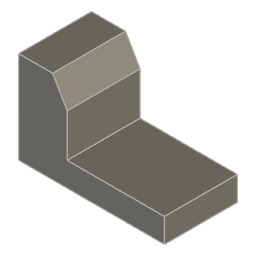
irtxcase (Autodesk Fusion 360 archive; units mm, degrees)
design "PCBMount - non-clip - 1mm"
Autodesk Fusion 360 part; units mm, degrees
note: some values were not read from the file. Chosen so that the rebuilt part matches the saved one: which face or edge a step refers to; which pieces of a blend or face edit are solid. Set by a fixed rule: which sketch regions a step uses.
sketch "Sketch1" plane through (0, 0, 0) normal (0, 1, 0) x (1, 0, 0)
  line L0 (0, 0) -> (6, 0)
  line L1 (6, 0) -> (6, -1)
  line L2 (6, -1) -> (2, -1)
  line L3 (2, -1) -> (2, -3.8)
  line L4 (2, -3.8) -> (0, -3.8)
  line L5 (0, -3.8) -> (0, 0)
  dimension "d1" = 2.8
  dimension "d2" = 1
  dimension "d3" = 2
  dimension "d4" = 4
  constraint coincident L0.start L5.end
  constraint horizontal L0
  constraint perpendicular L0 L1
  constraint perpendicular L1 L2
  constraint perpendicular L2 L3
  constraint perpendicular L4 L5
  constraint coincident L3.end L4.start
  measures "d1" distance of L2.end L3.end
  measures "d2" distance of L0.end L1.end
  measures "d3" distance of L3 L5
  measures "d4" distance of L1 L3
extrude "Extrude1" add sketch "Sketch1" along normal blind 3
sketch "Sketch4" plane through (0, 0, 0) normal (0, 0, -1) x (1, 0, 0)
  line L0 (6, 0) -> (0, 0)
  line L1 (0, 0) -> (0, -3)
  line L2 (0, -3) -> (6, -3)
  line L3 (6, -3) -> (6, 0)
  line L4 (0, -1.5) -> (6, -1.5) construction
  line L5 (2, 0) -> (2, -3) construction
  point P0 (2, -1.5)
  constraint midpoint L1 L4.start
  constraint midpoint L3 L4.end
  constraint midpoint L5 P0
chamfer "Chamfer3" distance 0.6 angle 60 1 edges at (2, 1.5, 3.8) measured on face at (1.3333, 1, 3.8)

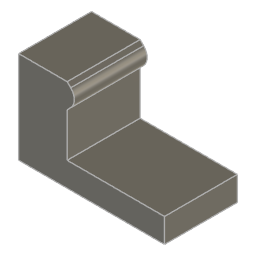
design "PCBMount - 1mm"
Autodesk Fusion 360 part; units mm, degrees
sketch "Sketch1" plane through (0, 0, 0) normal (0, 1, 0) x (1, 0, 0)
  line L0 (0, 0) -> (6, 0)
  line L1 (6, 0) -> (6, -1)
  line L2 (6, -1) -> (2, -1)
  line L3 (2, -1) -> (2, -2.8)
  line L4 (2, -2.8) -> (2.5, -2.8)
  line L5 (2.5, -2.8) -> (2.5, -3.8)
  line L6 (2.5, -3.8) -> (0, -3.8)
  line L7 (0, -3.8) -> (0, 0)
  dimension "d1" = 1.8
  dimension "d2" = 1
  dimension "d3" = 2
  dimension "d4" = 4
  dimension "d5" = 1
  dimension "d6" = 0.5
  constraint coincident L0.start L7.end
  constraint horizontal L0
  constraint perpendicular L0 L1
  constraint perpendicular L1 L2
  constraint perpendicular L2 L3
  constraint perpendicular L3 L4
  constraint perpendicular L4 L5
  constraint perpendicular L5 L6
  constraint perpendicular L6 L7
  measures "d1" distance of L2.end L3.end
  measures "d2" distance of L0.end L1.end
  measures "d3" distance of L3 L7
  measures "d4" distance of L1 L3
  measures "d5" distance of L4.end L5.end
  measures "d6" distance of L3 L5
extrude "Extrude1" add sketch "Sketch1" along normal blind 3
sketch "Sketch2" plane through (0, 0, 1) normal (0, 0, 1) x (-1, 0, 0)
  line L0 (-2, 0) -> (-6, 0)
  line L1 (-6, 0) -> (-6, -3)
  line L2 (-6, -3) -> (-2, -3)
  line L3 (-2, -3) -> (-2, 0)
  line L4 (0, 0) -> (0, -3) construction
  line L5 (-6, -1.5) -> (0, -1.5) construction
  line L6 (-4.5, -3) -> (-4.5, 0) construction
  line L7 (-6, 0) -> (-2, 0) construction
  circle A0 centre (-4.5, -1.5) radius 1.25
  dimension "d9" = 1.5
  dimension "d10" = 1.5
  dimension "d11" = 2.5
  dimension "d15" = 2.5
  constraint midpoint L1 L5.start
  constraint midpoint L4 L5.end
  constraint coincident L2 L6.start
  constraint coincident L0 L6.end
  constraint perpendicular L6 L7
  constraint midpoint L6 A0.centre
  measures "d9" distance of L5 L7
  measures "d10" distance of L1 L6
  measures "d11" diameter of A0
  measures "d15" distance of L3 L6
chamfer "Chamfer2" distance 0.5 angle 45 2 edges at (2.5, 1.5, 2.8) (2.5, 1.5, 3.8)
fillet "Fillet1" radius 0.5 4 edges at (2.5, 0, 3.3) (2.5, 1.5, 3.2999) (2.5, 3, 3.3) (2.5, 1.5, 3.3001)
sketch "Sketch4" plane through (0, 0, 0) normal (0, 0, -1) x (1, 0, 0)
  line L0 (6, 0) -> (0, 0)
  line L1 (0, 0) -> (0, -3)
  line L2 (0, -3) -> (6, -3)
  line L3 (6, -3) -> (6, 0)
  line L4 (0, -1.5) -> (6, -1.5) construction
  line L5 (2, 0) -> (2, -3) construction
  point P0 (2, -1.5)
  constraint midpoint L1 L4.start
  constraint midpoint L3 L4.end
  constraint midpoint L5 P0
equation "d10 = d9"

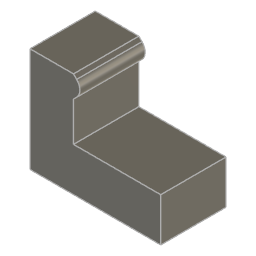
design "PCBMount"
Autodesk Fusion 360 part; units mm, degrees
sketch "Sketch1" plane through (0, 0, 0) normal (0, 1, 0) x (1, 0, 0)
  line L0 (0, 0) -> (6, 0)
  line L1 (6, 0) -> (6, -2)
  line L2 (6, -2) -> (2, -2)
  line L3 (2, -2) -> (2, -3.8)
  line L4 (2, -3.8) -> (2.5, -3.8)
  line L5 (2.5, -3.8) -> (2.5, -4.8)
  line L6 (2.5, -4.8) -> (0, -4.8)
  line L7 (0, -4.8) -> (0, 0)
  dimension "d1" = 1.8
  dimension "d2" = 2
  dimension "d3" = 2
  dimension "d4" = 4
  dimension "d5" = 1
  dimension "d6" = 0.5
  constraint coincident L0.start L7.end
  constraint horizontal L0
  constraint perpendicular L0 L1
  constraint perpendicular L1 L2
  constraint perpendicular L2 L3
  constraint perpendicular L3 L4
  constraint perpendicular L4 L5
  constraint perpendicular L5 L6
  constraint perpendicular L6 L7
  measures "d1" distance of L2.end L3.end
  measures "d2" distance of L0.end L1.end
  measures "d3" distance of L3 L7
  measures "d4" distance of L1 L3
  measures "d5" distance of L4.end L5.end
  measures "d6" distance of L3 L5
extrude "Extrude1" add sketch "Sketch1" along normal blind 3
sketch "Sketch2" plane through (0, 0, 2) normal (0, 0, 1) x (-1, 0, 0)
  line L0 (-2, 0) -> (-6, 0)
  line L1 (-6, 0) -> (-6, -3)
  line L2 (-6, -3) -> (-2, -3)
  line L3 (-2, -3) -> (-2, 0)
  line L4 (0, 0) -> (0, -3) construction
  line L5 (-6, -1.5) -> (0, -1.5) construction
  line L6 (-4.5, -3) -> (-4.5, 0) construction
  line L7 (-6, 0) -> (-2, 0) construction
  circle A0 centre (-4.5, -1.5) radius 1.25
  dimension "d9" = 1.5
  dimension "d10" = 1.5
  dimension "d11" = 2.5
  dimension "d15" = 2.5
  constraint midpoint L1 L5.start
  constraint midpoint L4 L5.end
  constraint coincident L2 L6.start
  constraint coincident L0 L6.end
  constraint perpendicular L6 L7
  constraint midpoint L6 A0.centre
  measures "d9" distance of L5 L7
  measures "d10" distance of L1 L6
  measures "d11" diameter of A0
  measures "d15" distance of L3 L6
chamfer "Chamfer2" distance 0.5 angle 45 2 edges at (2.5, 1.5, 3.8) (2.5, 1.5, 4.8)
fillet "Fillet1" radius 0.5 4 edges at (2.5, 0, 4.3) (2.5, 1.5, 4.2999) (2.5, 3, 4.3) (2.5, 1.5, 4.3001)
sketch "Sketch4" plane through (0, 0, 0) normal (0, 0, -1) x (1, 0, 0)
  line L0 (6, 0) -> (0, 0)
  line L1 (0, 0) -> (0, -3)
  line L2 (0, -3) -> (6, -3)
  line L3 (6, -3) -> (6, 0)
  line L4 (0, -1.5) -> (6, -1.5) construction
  line L5 (2, 0) -> (2, -3) construction
  point P0 (2, -1.5)
  constraint midpoint L1 L4.start
  constraint midpoint L3 L4.end
  constraint midpoint L5 P0
equation "d10 = d9"
